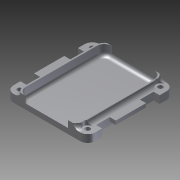
# Autodesk Inventor part: x-IMU Calibration Cube Bracket
Saved by Autodesk Inventor 2011 (Build 150239000, 239)
## iProperties
Created: 2011-08-25
Part Number: x-IMU Calibration Cube Bracket
Document SubType Name: Modeling
Designer: Seb Madgwick
Density: 1 g/cm^3
Author: Seb Madgwick
Autodesk Inventor part; units mm, degrees
ref_plane "YZ Plane" through (0, 0, 0) normal (1, 0, 0) x (0, 1, 0)
ref_plane "XZ Plane" through (0, 0, 0) normal (0, 1, 0) x (-1, 0, 0)
ref_plane "XY Plane" through (0, 0, 0) normal (0, 0, 1) x (1, 0, 0)
sketch "Sketch2" plane through (0, 0, 0) normal (0, 1, 0) x (-1, 0, 0)
  line L0 (22, -29.5) -> (-22, -29.5)
  line L1 (-27, -24.5) -> (-27, 24.5)
  line L2 (-22, 29.5) -> (22, 29.5)
  line L3 (27, 24.5) -> (27, -24.5)
  arc A0 (27, 24.5) -> (22, 29.5) centre (22, 24.5) ccw
  arc A1 (22, -29.5) -> (27, -24.5) centre (22, -24.5) ccw
  arc A2 (-22, 29.5) -> (-27, 24.5) centre (-22, 24.5) ccw
  arc A3 (-27, -24.5) -> (-22, -29.5) centre (-22, -24.5) ccw
  point P0 (0, 0)
  point P1 (27, -29.5)
  point P2 (-27, 29.5)
  point P3 (-27, -29.5)
  point P4 (27, 29.5)
  point P5 (27, 0)
  point P6 (0, -29.5)
  dimension "d0" = 54
  dimension "d1" = 59
  dimension "d14" = 5
  constraints: 8 end point, 8 point on circle, 8 point on line, 8 tangent, 4 centre point, 3 equal radius, 2 midpoint, 2 parallel, 1 horizontal, 1 horizontal alignment, 1 perpendicular, 1 vertical alignment
  measures "d0" distance of point (27, -29.5) point (-27, -29.5)
  measures "d1" distance of point (27, 29.5) point (27, -29.5)
  measures "d14" radius of A0
extrude "Extrusion_main" add sketch "Sketch2" along normal blind 5
sketch "Sketch4" plane through (0, 5, 0) normal (0, 1, 0) x (1, 0, 0)
  line L0 (-14, 28.5) -> (14, 28.5)
  line L1 (19, 23.5) -> (19, -23.5)
  line L2 (14, -28.5) -> (-14, -28.5)
  line L3 (-19, -23.5) -> (-19, 23.5)
  arc A0 (19, 23.5) -> (14, 28.5) centre (14, 23.5) ccw
  arc A1 (14, -28.5) -> (19, -23.5) centre (14, -23.5) ccw
  arc A2 (-19, -23.5) -> (-14, -28.5) centre (-14, -23.5) ccw
  arc A3 (-14, 28.5) -> (-19, 23.5) centre (-14, 23.5) ccw
  point P0 (0, 0)
  point P1 (-19, 28.5)
  point P2 (19, -28.5)
  point P3 (19, 28.5)
  point P4 (19, 0)
  point P5 (0, 28.5)
  dimension "d9" = 57
  dimension "d10" = 38
  dimension "d11" = 5
  constraints: 8 end point, 8 point on circle, 8 tangent, 6 point on line, 4 centre point, 3 equal radius, 2 midpoint, 2 parallel, 1 horizontal, 1 horizontal alignment, 1 perpendicular, 1 vertical alignment
  measures "d9" distance of point (19, 28.5) point (19, -28.5)
  measures "d10" distance of point (-19, 28.5) point (19, 28.5)
  measures "d11" radius of A0
extrude "Extrusion_dockingRecess" cut sketch "Sketch4" against normal blind 4
fillet "Fillet_bottomFilit" radius 2.5 8 edges at (-19, 1, 0) (-17.5355, 1, 27.0355) (0, 1, 28.5) (17.5355, 1, 27.0355) (19, 1, 0) (17.5355, 1, -27.0355) (0, 1, -28.5) (-17.5355, 1, -27.0355)
sketch "Sketch5" plane through (0, 5, 0) normal (0, 1, 0) x (1, 0, 0)
  arc A0 (-14, 28.5) -> (-19, 23.5) centre (-14, 23.5) ccw projected
  line L0 (-14, 28.5) -> (14, 28.5) projected
  arc A1 (19, 23.5) -> (14, 28.5) centre (14, 23.5) ccw projected
  line L1 (19, 23.5) -> (19, -23.5) projected
  arc A2 (14, -28.5) -> (19, -23.5) centre (14, -23.5) ccw projected
  line L2 (14, -28.5) -> (-14, -28.5) projected
  arc A3 (-19, -23.5) -> (-14, -28.5) centre (-14, -23.5) ccw projected
  line L3 (-19, -23.5) -> (-19, 23.5) projected
  line L4 (22, -29.5) -> (-22, -29.5) projected
  line L5 (-14, -29.5) -> (14, -29.5)
  arc A4 (14, -29.5) -> (20, -23.5) centre (14, -23.5) ccw
  line L6 (20, -23.5) -> (20, 23.5)
  arc A5 (20, 23.5) -> (14, 29.5) centre (14, 23.5) ccw
  line L7 (14, 29.5) -> (-14, 29.5)
  arc A6 (-14, 29.5) -> (-20, 23.5) centre (-14, 23.5) ccw
  line L8 (-20, 23.5) -> (-20, -23.5)
  arc A7 (-20, -23.5) -> (-14, -29.5) centre (-14, -23.5) ccw
  point P0 (0, 0)
  constraints: 8 end point, 8 point on circle, 4 centre point, 1 collinear, 7 other
extrude "Extrusion_wall" add sketch "Sketch5" along normal blind 3
fillet "Fillet_wallSupport" radius 3 6 edges at (20, 5, 0) (18.2426, 5, 27.7426) (18.2426, 5, -27.7426) (-20, 5, 0) (-18.2426, 5, -27.7426) (-18.2426, 5, 27.7426)
sketch "Sketch6" plane through (0, 0, 0) normal (0, -1, 0) x (1, 0, 0)
  circle A0 centre (22.5, 24) radius 1.55
  point P0 (0, 0)
  dimension "d20" = 22.5
  dimension "d21" = 24
  dimension "d27" = 3.1
  constraints: 1 centre point
  measures "d20" horizontal distance of point (0, 0) A0.centre
  measures "d21" vertical distance of point (0, 0) A0.centre
  measures "d27" diameter of A0
extrude "Extrusion_hole" cut sketch "Sketch6" against normal through all
sketch "Sketch7" plane through (0, 5, 0) normal (0, 1, 0) x (1, 0, 0)
  arc A0 (22.7689, -25.5265) -> (23, -22.5329) centre (22.5, -24) ccw projected
  circle A1 centre (22.5, -24) radius 3
  point P0 (0, 0)
  dimension "d24" = 6
  constraints: 1 centre point, 1 coincident
  measures "d24" diameter of A1
extrude "Extrusion_holeClearance" cut sketch "Sketch7" along normal through all
mirror "Mirror_holeRight" about plane through (0, 0, 0) normal (0, 0, 1) of "Extrusion_holeClearance", "Extrusion_hole"
mirror "Mirror_holesLeft" about plane through (0, 0, 0) normal (1, 0, 0) of "Extrusion_holeClearance", "Extrusion_hole", "Mirror_holeRight"
sketch "Sketch8" plane through (27, 0, 24.5) normal (1, 0, 0) x (0, 0, -1)
  line L0 (49, 0) -> (0, 0) projected
  line L1 (5.5, 5) -> (5.5, 0)
  line L2 (34.5, 5) -> (34.5, 2.5)
  line L3 (34.5, 2.5) -> (14.5, 2.5)
  line L4 (14.5, 2.5) -> (14.5, 5)
  line L5 (43.5, 5) -> (43.5, 0)
  line L6 (5.5, 5) -> (14.5, 5)
  line L7 (34.5, 5) -> (43.5, 5)
  line L8 (5.5, 0) -> (43.5, 0)
  point P0 (24.5, 0)
  point P1 (24.5, 5)
  point P2 (24.5, 0)
  dimension "d33" = 20
  dimension "d34" = 2.5
  dimension "d35" = 19
  dimension "d36" = 19
  constraints: 16 end point, 3 perpendicular, 2 parallel, 2 point on line, 1 collinear, 1 midpoint, 1 vertical alignment
  measures "d33" distance of L4.end L2.start
  measures "d34" distance of L3.end L4.end
  measures "d35" distance from line of L1 point (24.5, 0)
  measures "d36" distance from line of L5 point (24.5, 0)
extrude "Extrusion_strapNotches" cut sketch "Sketch8" against normal blind 4
mirror "Mirror_strapNotches" about plane through (0, 0, 0) normal (1, 0, 0) of "Extrusion_strapNotches"
sketch "Sketch9" plane through (0, 0, 0) normal (0, -1, 0) x (1, 0, 0)
  line L0 (27, -24.5) -> (27, -19) projected
  circle A0 centre (22.5, 24) radius 1.55 projected
  circle A1 centre (22.5, -24) radius 1.55 projected
  circle A2 centre (-22.5, 24) radius 1.55 projected
  circle A3 centre (-22.5, -24) radius 1.55 projected
  line L1 (22, 28.5) -> (-22, 28.5)
  line L2 (-27, 23.5) -> (-27, -23.5)
  line L3 (-22, -28.5) -> (22, -28.5)
  line L4 (27, -23.5) -> (27, 23.5)
  arc A4 (27, 23.5) -> (22, 28.5) centre (22, 23.5) ccw
  arc A5 (22, -28.5) -> (27, -23.5) centre (22, -23.5) ccw
  arc A6 (-27, -23.5) -> (-22, -28.5) centre (-22, -23.5) ccw
  arc A7 (-22, 28.5) -> (-27, 23.5) centre (-22, 23.5) ccw
  point P0 (0, 0)
  point P1 (27, 0)
  point P2 (0, -28.5)
  dimension "d39" = 5
  dimension "d40" = 57
  constraints: 8 end point, 8 point on circle, 8 tangent, 4 centre point, 3 equal radius, 2 midpoint, 2 parallel, 1 collinear, 1 horizontal, 1 horizontal alignment, 1 perpendicular, 1 vertical alignment
  measures "d39" radius of A4
  measures "d40" distance between parallel lines of L3 L1
extrude "Extrusion_finalMask" cut sketch "Sketch9" against normal through all keep common part
equation "\"d36\" = d35"
body "Solid1"
